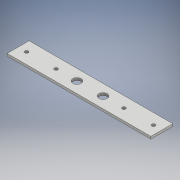
# Autodesk Inventor part: Drivetrainsideoutside
Saved by Autodesk Inventor 2017 (Build 210142000, 142)
## iProperties
Created: 2016-10-18
Part Number: Drivetrainsideoutside
Material: Generic
Document SubType Name: Sheet Metal
Designer: aesen
Density: 1 g/cm^3
Sheet Metal Rule: Default_mm
Appearance: Default
Author: aesen
Autodesk Inventor part; units mm, degrees
ref_plane "YZ Plane" through (0, 0, 0) normal (1, 0, 0) x (0, 1, 0)
ref_plane "XZ Plane" through (0, 0, 0) normal (0, 1, 0) x (-1, 0, 0)
ref_plane "XY Plane" through (0, 0, 0) normal (0, 0, 1) x (1, 0, 0)
sketch "Sketch1" plane through (0, 0, 0) normal (0, 0, 1) x (1, 0, 0)
  line L0 (-275.4315, -42) -> (-275.4315, 42)
  line L1 (-275.4315, 42) -> (3.3922, 42)
  line L2 (-275.4315, -42) -> (3.414, -42)
  circle A0 centre (243.4082, 0) radius 6.35
  circle A1 centre (50.0126, 0) radius 15.875
  circle A2 centre (130.1242, 0) radius 6.35
  line L3 (275.4315, -42) -> (3.414, -42)
  line L4 (275.4315, 42) -> (3.3922, 42)
  line L5 (275.4315, -42) -> (275.4315, 42)
  circle A3 centre (-50.0126, 0) radius 15.875
  circle A4 centre (-130.1242, 0) radius 6.35
  circle A5 centre (-243.4082, 0) radius 6.35
  point P0 (0.2172, 42)
  point P1 (0.2172, -42)
  dimension "d12" = 550.863
  dimension "d13" = 12.7
  dimension "d14" = 12.7
  dimension "d33" = 84
  dimension "d34" = 113.284
  dimension "d37" = 113.284
  dimension "d40" = 32.0233
  dimension "d44" = 12.7
  dimension "d45" = 12.7
  dimension "d48" = 32.0233
  dimension "d49" = 80.1116
  dimension "d50" = 100.0252
  constraints: 12 end point, 6 centre point, 2 point on line, 1 horizontal
  measures "d12" distance between parallel lines of L0 L5
  measures "d13" diameter of A2
  measures "d14" diameter of A0
  measures "d33" distance of L3.start L4.start
  measures "d34" distance of A0.centre A2.centre
  measures "d37" distance of A4.centre A5.centre
  measures "d40" distance from line of L0 A5.centre
  measures "d44" diameter of A4
  measures "d45" diameter of A5
  measures "d48" distance from line of L5 A0.centre
  measures "d49" distance of A2.centre A1.centre
  measures "d50" distance of A1.centre A3.centre
extrude "Extrusion3" add sketch "Sketch1" along normal blind 9.525
equation "\"BendRadius\" = Thickness"
equation "\"BendReliefWidth\" = Thickness"
equation "\"BendReliefDepth\" = 0.5 * Thickness"
equation "\"CornerReliefSize\" = 4 * Thickness"
equation "\"MinimumRemnant\" = 2 * Thickness"
equation "\"TransitionRadius\" = BendRadius"
equation "\"JacobiRadiusSize\" = BendRadius"
equation "\"GapSize\" = Thickness"
equation "\"Thickness\" = 0.5"
body "Solid3"
